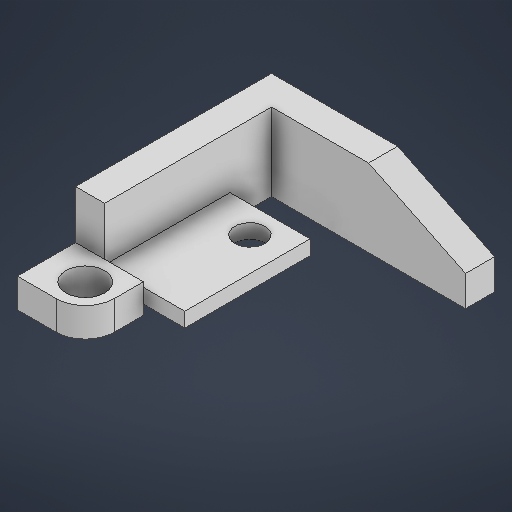
# Autodesk Inventor part: rfmw
Saved by Autodesk Inventor 2026.2 (Build 302298010, 298A)
## iProperties
Created: 2026-04-27
Part Number: rfmw
Material: Ogólny
Document SubType Name: Modeling
Designer: karol
Density: 1 g/cm^3
Appearance: Domyślna
Mass: 0.888 g
Surface Area: 8.70622 cm^2
Volume: 0.888 cm^3
Author: karol
Autodesk Inventor part; units mm, degrees
ref_plane "YZ Plane" through (0, 0, 0) normal (1, 0, 0) x (0, 1, 0)
ref_plane "XZ Plane" through (0, 0, 0) normal (0, 1, 0) x (-1, 0, 0)
ref_plane "XY Plane" through (0, 0, 0) normal (0, 0, 1) x (1, 0, 0)
sketch "Szkic1" plane through (0, 0, 0) normal (0, 1, 0) x (-1, 0, 0)
  line L0 (0, 0) -> (3, 0)
  line L1 (3, 0) -> (3, -22)
  line L2 (3, -22) -> (0, -22)
  line L3 (0, -22) -> (0, 0)
  line L4 (0, 0) -> (-3, 0)
  line L5 (-3, 0) -> (-3, -5)
  line L6 (-3, -5) -> (0, -5)
  line L7 (0, -5) -> (0, 0)
  line L8 (0, -22) -> (-20, -22)
  line L9 (-20, -22) -> (-20, -19)
  line L10 (-20, -19) -> (0, -19)
  line L11 (0, -19) -> (0, -22)
  dimension "d0" = 3
  dimension "d1" = 22
  dimension "d2" = 3
  dimension "d3" = 5
  dimension "d4" = 20
  dimension "d5" = 3
  constraints: 24 end point, 6 parallel, 3 horizontal, 3 perpendicular
  measures "d0" distance of L1.end L2.end
  measures "d1" distance of L0.end L1.end
  measures "d2" distance of L6.end L5.end
  measures "d3" distance of L5.end L4.end
  measures "d4" distance of L9.end L10.end
  measures "d5" distance of L8.end L9.end
extrude "Wyciągnięcie proste1" add sketch "Szkic1" along normal blind 8
sketch "Szkic2" plane through (0, 0, -19) normal (0, 0, 1) x (1, 0, 0)
  line L0 (20, 0) -> (20, 8) projected
  line L1 (20, 0) -> (0, 8)
  line L2 (20, 8) -> (-3, 8) projected
  point P0 (0, 0)
  constraints: 2 end point, 1 point on line
extrude "Wyciągnięcie proste2" cut sketch "Szkic2" against normal blind 3
sketch "Szkic3" plane through (-3, 0, 0) normal (0, 0, 1) x (1, 0, 0)
  line L0 (0, 0) -> (0, 8) projected
  line L1 (0, 0) -> (6, 0)
  line L2 (6, 0) -> (6, 8)
  line L3 (6, 8) -> (0, 8)
  line L4 (0, 8) -> (0, 0)
  point P0 (3, 0)
  constraints: 8 end point, 2 parallel, 1 horizontal, 1 perpendicular
extrude "Wyciągnięcie proste3" add sketch "Szkic3" along normal blind 4.2
sketch "Szkic4" plane through (3, 0, -5) normal (0, 0, -1) x (-1, 0, 0)
  line L0 (0, 0) -> (0, 8) projected
  line L1 (3, 0) -> (3, 8) projected
  line L2 (0, 8) -> (3, 8)
  line L3 (3, 8) -> (3, 0)
  line L4 (3, 0) -> (0, 0)
  line L5 (0, 0) -> (0, 8)
  constraints: 8 end point, 2 parallel, 1 horizontal, 1 perpendicular
extrude "Wyciągnięcie proste4" cut sketch "Szkic4" against normal blind 3.2
sketch "Szkic6" plane through (3, 0, 4.2) normal (1, 0, 0) x (0, 0, -1)
  line L0 (0, 8) -> (0, 0) projected
  line L1 (23.2, 0) -> (6, 0) projected
  line L2 (0, 8) -> (6, 8)
  line L3 (6, 8) -> (6, 0)
  line L4 (6, 0) -> (0, 0)
  line L5 (0, 0) -> (0, 8)
  point P0 (4.2, 0)
  constraints: 8 end point, 2 parallel, 1 horizontal, 1 perpendicular
extrude "Wyciągnięcie proste7" add sketch "Szkic6" along normal blind 2
sketch "Szkic7" plane through (0, 8, 0) normal (0, 1, 0) x (1, 0, 0)
  circle A0 centre (1, -1.2) radius 2
  line L0 (5, 1.8) -> (5, -4.2) projected
  line L1 (-3, -4.2) -> (5, -4.2) projected
  line L2 (-3, 22) -> (-3, -4.2) projected
  line L3 (5, -4.2) -> (-3, -4.2)
  line L4 (-3, -4.2) -> (-3, 1.8)
  line L5 (-3, 1.8) -> (5, 1.8)
  line L6 (5, 1.8) -> (5, -4.2)
  point P0 (0, 0)
  dimension "d23" = 4
  dimension "d24" = 4
  dimension "d25" = 3
  constraints: 8 end point, 2 parallel, 1 centre point, 1 horizontal, 1 perpendicular, 1 point on line
  measures "d23" diameter of A0
  measures "d24" distance from line of L0 A0.centre
  measures "d25" distance from line of L1 A0.centre
extrude "Wyciągnięcie proste8" cut sketch "Szkic7" against normal blind 8 contours A0
extrude "Wyciągnięcie proste9" cut sketch "Szkic7" against normal blind 5 contours A0 | L0 L1 L2 L5
sketch "Szkic8" plane through (5, 0, 4.2) normal (1, 0, 0) x (0, 0, -1)
  line L0 (0, 3) -> (0, 0) projected
  line L1 (23.2, 0) -> (6, 0) projected
  line L2 (0, 3) -> (6, 3)
  line L3 (6, 3) -> (6, 0)
  line L4 (6, 0) -> (0, 0)
  line L5 (0, 0) -> (0, 3)
  point P0 (4.2, 0)
  constraints: 8 end point, 2 parallel, 1 horizontal, 1 perpendicular
extrude "Wyciągnięcie proste10" cut sketch "Szkic8" against normal blind 1
sketch "Szkic9" plane through (-3, 0, -22) normal (0, 0, -1) x (-1, 0, 0)
  line L0 (-3, 8) -> (-23, 0) projected
  line L1 (-23, 0) -> (-23, 3.137)
  line L2 (-3, 8) -> (-13, 8)
  line L3 (-13, 8) -> (-23, 3.137)
  point P0 (-3, 0)
  dimension "d32" = 3.137
  constraints: 6 end point, 1 horizontal, 1 vertical
  measures "d32" distance of L0.end L1.end
extrude "Wyciągnięcie proste11" add sketch "Szkic9" against normal blind 3
sketch "Szkic10" plane through (0, 0, -19) normal (1, 0, 0) x (0, 0, -1)
  line L0 (0, 0) -> (-17.2, 0) projected
  line L1 (-17.2, 0) -> (-4.28, 0)
  line L2 (-4.28, 0) -> (-4.28, 1.5)
  line L3 (-4.28, 1.5) -> (-17.2, 1.5)
  line L4 (-17.2, 1.5) -> (-17.2, 0)
  point P0 (-19, 0)
  point P1 (-4.28, 0)
  dimension "d35" = 12.92
  dimension "d36" = 1.5
  constraints: 8 end point, 2 parallel, 1 horizontal, 1 perpendicular
  measures "d35" distance of L3.end L2.end
  measures "d36" distance of L2.end L1.end
extrude "Wyciągnięcie proste12" add sketch "Szkic10" along normal blind 8.26
sketch "Szkic11" plane through (0, 1.5, -1.8) normal (0, 1, 0) x (1, 0, 0)
  circle A0 centre (4.8, 10.17) radius 1.55
  line L0 (4, 0) -> (8.26, 0) projected
  line L1 (0, 0) -> (0, 17.2) projected
  point P0 (0, -1.8)
  dimension "d39" = 3.1
  dimension "d40" = 10.17
  dimension "d41" = 4.8
  constraints: 1 centre point
  measures "d39" diameter of A0
  measures "d40" distance from line of L0 A0.centre
  measures "d41" distance from line of L1 A0.centre
extrude "Wyciągnięcie proste13" cut sketch "Szkic11" against normal blind 2
fillet "Fillet1" radius 3 1 edges at (4, 1.5, 4.2)
sketch "Szkic12" plane through (0, 1.5, -1.8) normal (0, 1, 0) x (1, 0, 0)
  circle A0 centre (4.8, 10.17) radius 1.55 projected
  line L0 (0, 0) -> (0, 12.92) projected
  line L1 (4, 0) -> (0, 0) projected
  line L2 (4, 0) -> (8.26, 0) projected
  line L3 (8.26, 12.92) -> (8.26, 0) projected
  line L4 (0, 12.92) -> (8.26, 12.92) projected
  point P0 (0, -1.8)
extrude "Wyciągnięcie proste14" add sketch "Szkic12" along normal blind 1
sketch "Szkic13" plane through (0, 0, 0) normal (0, -1, 0) x (1, 0, 0)
  line L0 (8.26, -1.8) -> (8.26, -14.72) projected
  line L1 (8.26, -14.72) -> (0, -14.72) projected
  line L2 (0, -1.8) -> (0, -14.72) projected
  line L3 (4, -1.8) -> (0, -1.8) projected
  line L4 (4, -1.8) -> (8.26, -1.8) projected
  circle A0 centre (4.8, -11.97) radius 1.55 projected
  point P0 (0, 0)
extrude "Wyciągnięcie proste15" cut sketch "Szkic13" against normal blind 1
